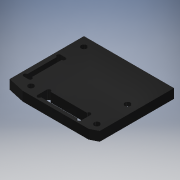
# Autodesk Inventor part: コックピット_サブフレーム_1_5
Saved by Autodesk Inventor 2018 (Build 220112000, 112)
## iProperties
Created: 2016-05-09
Part Number: コックピット_サブフレーム_1_5
Material: アセタール樹脂、黒
Document SubType Name: Modeling
Designer: hiroaki
Density: 1.425 g/cm^3
Appearance: 滑らか - 黒
Mass: 4.98887 g
Surface Area: 48.5671 cm^2
Volume: 3.50096 cm^3
Author: hiroaki
Autodesk Inventor part; units mm, degrees
ref_plane "YZ Plane" through (0, 0, 0) normal (1, 0, 0) x (0, 1, 0)
ref_plane "XZ Plane" through (0, 0, 0) normal (0, 1, 0) x (-1, 0, 0)
ref_plane "XY Plane" through (0, 0, 0) normal (0, 0, 1) x (1, 0, 0)
sketch "スケッチ1" plane through (0, 0, 0) normal (0, 0, 1) x (1, 0, 0)
  line L0 (-24.25, -20) -> (24.25, -20) construction
  line L1 (24.25, -20) -> (24.25, 20)
  line L2 (24.25, 20) -> (-24.25, 20)
  line L3 (-24.25, 20) -> (-24.25, -20)
  line L4 (-24.25, -20) -> (24.25, 20) construction
  line L5 (24.25, -20) -> (-24.25, 20) construction
  circle A0 centre (-15.25, -17.5) radius 1.55
  circle A1 centre (20.25, -17.5) radius 1.55
  line L6 (-9.25, -15) -> (14.25, -15) construction
  line L7 (14.25, -15) -> (14.25, -20) construction
  line L8 (14.25, -20) -> (-9.25, -20) construction
  line L9 (-9.25, -20) -> (-9.25, -15) construction
  line L10 (-24.25, -20) -> (-15.25, -22)
  line L11 (-15.25, -22) -> (20.25, -22)
  line L12 (20.25, -22) -> (24.25, -20)
  line L13 (14.3, -14.95) -> (-9.3, -14.95)
  line L14 (-9.3, -14.95) -> (-9.3, -20.05)
  line L15 (-9.3, -20.05) -> (14.3, -20.05)
  line L16 (14.3, -20.05) -> (14.3, -14.95)
  circle A2 centre (-8.25, -14.95) radius 1.05
  circle A3 centre (-8.25, -20.05) radius 1.05
  circle A4 centre (13.25, -14.95) radius 1.05
  circle A5 centre (13.25, -20.05) radius 1.05
  circle A6 centre (-19.25, 15) radius 1.55
  line L17 (-21.8, 5.05) -> (-19.2, 5.05)
  line L18 (-19.2, 5.05) -> (-19.2, -15.05)
  line L19 (-19.2, -15.05) -> (-21.8, -15.05)
  line L20 (-21.8, -15.05) -> (-21.8, 5.05)
  line L21 (-19.25, 5) -> (-21.75, 5) construction
  line L22 (-21.75, 5) -> (-21.75, -15) construction
  line L23 (-21.75, -15) -> (-19.25, -15) construction
  line L24 (-19.25, -15) -> (-19.25, 5) construction
  line L25 (2.5, -14.95) -> (2.5, -20.05) construction
  circle A7 centre (19.25, 0) radius 1.55
  line L26 (-19.25, 15) -> (19.25, 15) construction
  line L27 (19.25, 15) -> (19.25, 0) construction
  circle A8 centre (-21.8, 4) radius 1.05
  circle A9 centre (-19.2, 4) radius 1.05
  circle A10 centre (-21.8, -14) radius 1.05
  circle A11 centre (-19.2, -14) radius 1.05
  point P0 (0, 0)
  point P1 (-9.25, -17.5)
  dimension "d10" = 2.1
  dimension "d26" = 2.1
  dimension "d0" = 5
  dimension "d3" = 3.1
  dimension "d4" = 35.5
  dimension "d5" = 2
  dimension "d7" = 40
  dimension "d8" = 23.5
  dimension "d9" = 0.05
  dimension "d11" = 3.1
  dimension "d12" = 5
  dimension "d13" = 5
  dimension "d14" = 0.05
  dimension "d15" = 17.75
  dimension "d16" = 48.5
  dimension "d17" = 4
  dimension "d18" = 5
  dimension "d19" = 20
  dimension "d20" = 2.5
  dimension "d21" = 2.5
  dimension "d22" = 5
  dimension "d23" = 15
  dimension "d27" = 25
  constraints: 56 end point, 10 parallel, 8 point on line, 6 horizontal alignment, 6 perpendicular, 6 vertical alignment, 5 midpoint, 4 centre point, 4 horizontal, 2 equal radius, 1 collinear, 22 other
  measures "d0" distance of L8.end L6.start
  measures "d3" diameter of A0
  measures "d4" distance of A1.centre A0.centre
  measures "d5" distance between parallel lines of L11 L0
  measures "d7" distance of L0.end L1.end
  measures "d8" distance of L6.start L6.end
  measures "d9" distance between parallel lines of L13 L6
  measures "d11" diameter of A6
  measures "d12" distance from line of L3 L26.start
  measures "d13" distance from line of L2 L26.start
  measures "d14" distance between parallel lines of L17 L21
  measures "d15" distance from line of A0.centre L25
  measures "d16" distance of L1.end L2.end
  measures "d17" distance from line of L1 A1.centre
  measures "d18" distance between parallel lines of L1 L27
  measures "d19" distance from line of L2 L27.end
  measures "d20" distance of L21.start L21.end
  measures "d21" distance between parallel lines of L22 L3
  measures "d22" distance between parallel lines of L23 L0
  measures "d23" distance between parallel lines of L2 L21
  measures "d27" distance between parallel lines of L21 L0
extrude "押し出し1" add sketch "スケッチ1" along normal blind 5
sketch "スケッチ2" plane through (0, 0, 0) normal (0, 0, -1) x (-1, 0, 0)
  line L0 (-14.3, -20.05) -> (-14.3, -14.95) projected
  line L1 (-12.2, -14.95) -> (7.2, -14.95) projected
  line L2 (24.25, 20) -> (-24.25, 20) projected
  line L3 (-24.25, 20) -> (-24.25, -20) projected
  line L4 (21.8, -15.05) -> (19.2, -15.05) projected
  line L5 (19.2, -12.95) -> (19.2, 2.95) projected
  line L6 (19.2, 5.05) -> (21.8, 5.05) projected
  line L7 (-20.25, 16) -> (16.25, 16)
  line L8 (16.25, 16) -> (16.25, -11)
  line L9 (16.25, -11) -> (-20.25, -11)
  line L10 (-20.25, -11) -> (-20.25, -2.8284)
  line L11 (-20.25, 16) -> (-20.25, 2.8284)
  line L12 (19.25, 5.05) -> (19.25, -15.05) construction
  line L13 (19.2, -15.05) -> (21.8, -15.05) projected
  line L14 (-14.3, -15) -> (9.3, -15) construction
  line L15 (9.3, -20.05) -> (9.3, -14.95) projected
  arc A0 (-20.25, 2.8284) -> (-20.25, -2.8284) centre (-19.25, 0) ccw
  point P0 (0, 0)
  dimension "d29" = 4
  dimension "d30" = 4
  dimension "d31" = 0.05
  dimension "d32" = 3
  dimension "d33" = 0.05
  dimension "d34" = 4
  constraints: 14 end point, 4 point on line, 3 perpendicular, 2 horizontal, 2 point on circle, 2 vertical, 1 centre point, 1 vertical alignment
  measures "d29" distance between parallel lines of L3 L11
  measures "d30" distance between parallel lines of L2 L7
  measures "d31" distance between parallel lines of L12 L5
  measures "d32" distance between parallel lines of L8 L12
  measures "d33" distance between parallel lines of L1 L14
  measures "d34" distance between parallel lines of L14 L9
extrude "押し出し2" cut sketch "スケッチ2" against normal blind 3
fillet "フィレット1" radius 2 6 edges at (20.25, 2.8284, 1.5) (20.25, -2.8284, 1.5) (20.25, 16, 1.5) (-16.25, 16, 1.5) (-16.25, -11, 1.5) (20.25, -11, 1.5)
sketch "スケッチ3" plane through (0, 0, 0) normal (0, 0, -1) x (-1, 0, 0)
  circle A0 centre (15.25, -17.5) radius 1.55 projected
  circle A1 centre (15.25, -17.5) radius 3
  circle A2 centre (19.25, 15) radius 1.55 projected
  circle A3 centre (19.25, 15) radius 3
  circle A4 centre (-20.25, -17.5) radius 3
  point P0 (0, 0)
  dimension "d38" = 6
  dimension "d39" = 6
  dimension "d40" = 6
  constraints: 3 centre point, 2 coincident
  measures "d38" diameter of A1
  measures "d39" diameter of A3
  measures "d40" diameter of A4
extrude "押し出し3" cut sketch "スケッチ3" against normal blind 3.5
sketch "スケッチ5" plane through (0, 0, 0) normal (0, 0, -1) x (-1, 0, 0)
  line L0 (-18.25, 16) -> (14.25, 16) projected
  line L1 (14.25, 16) -> (16.4216, 16)
  circle A0 centre (19.25, 15) radius 3 projected
  line L2 (19.25, 12) -> (16.25, 12)
  line L3 (16.25, 14) -> (16.25, -9) projected
  line L4 (16.25, 14) -> (16.25, 12)
  arc A1 (16.25, 14) -> (14.25, 16) centre (14.25, 14) ccw
  arc A2 (16.4216, 16) -> (19.25, 12) centre (19.25, 15) ccw
  point P0 (0, 0)
  constraints: 6 end point, 6 point on circle, 2 centre point, 1 coincident, 1 horizontal, 1 parallel, 1 perpendicular, 1 point on line
extrude "押し出し4" cut sketch "スケッチ5" against normal blind 3 contours L1 A0 L2 L3 A1
fillet "フィレット2" radius 2 2 edges at (-16.4216, 16, 1.5) (-16.25, 12, 1.5)
equation "\"d13\" = d12"
equation "\"d15\" = 0.5 * d4"
equation "\"d18\" = d13"
